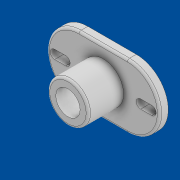
# Autodesk Inventor part: 부품1
Saved by Autodesk Inventor 2022 (Build 260153000, 153)
## iProperties
Created: 2022-09-19
Part Number: 부품1
Material: 일반
Document SubType Name: Modeling
Designer: USER
Density: 1 g/cm^3
Appearance: 기본값
Author: USER
Autodesk Inventor part; units mm, degrees
ref_plane "YZ Plane" through (0, 0, 0) normal (1, 0, 0) x (0, 1, 0)
ref_plane "XZ Plane" through (0, 0, 0) normal (0, 1, 0) x (-1, 0, 0)
sketch "스케치1" plane through (0, 0, 0) normal (0, 0, 1) x (1, 0, 0)
  line L0 (-22, 0) -> (22, 0) construction
  line L1 (-22, -29) -> (22, -29)
  line L2 (22, 29) -> (-22, 29)
  arc A0 (-22, 29) -> (-22, -29) centre (-22, 0) ccw
  arc A1 (22, -29) -> (22, 29) centre (22, 0) ccw
  line L3 (-44, 0) -> (-34, 0) construction
  line L4 (-44, -4) -> (-34, -4)
  line L5 (-34, 4) -> (-44, 4)
  arc A2 (-44, 4) -> (-44, -4) centre (-44, 0) ccw
  arc A3 (-34, -4) -> (-34, 4) centre (-34, 0) ccw
  line L6 (44, 0) -> (34, 0) construction
  line L7 (44, 4) -> (34, 4)
  line L8 (34, -4) -> (44, -4)
  arc A4 (44, -4) -> (44, 4) centre (44, 0) ccw
  arc A5 (34, 4) -> (34, -4) centre (34, 0) ccw
  circle A6 centre (0, 0) radius 18.5
  circle A7 centre (0, 0) radius 11
  point P0 (-39, 0)
  point P1 (39, 0)
  dimension "d0" = 29
  dimension "d1" = 102
  dimension "d2" = 10
  dimension "d3" = 8
  dimension "d4" = 10
  dimension "d5" = 8
  dimension "d6" = 68
  dimension "d7" = 34
  dimension "d8" = 37
  dimension "d9" = 22
  constraints: 24 end point, 12 point on circle, 12 tangent, 8 centre point, 3 coincident, 3 horizontal, 3 midpoint, 3 parallel
  measures "d0" radius of A1
  measures "d2" distance of L3.end L3.start
  measures "d3" distance between parallel lines of L5 L4
  measures "d4" distance of L6.start L6.end
  measures "d5" distance between parallel lines of L7 L8
  measures "d6" distance of L6.end L3.end
  measures "d7" distance of point (0, 0) L3.end
  measures "d8" diameter of A6
  measures "d9" diameter of A7
extrude "돌출1" add sketch "스케치1" along normal blind 8 contours A0 L2 A1 L1
extrude "돌출2" add sketch "스케치1" along normal blind 40 contours A6
ref_plane "작업 평면1" through (-22, 0, 0) normal (0, 1, 0) x (1, 0, 0)
sketch "스케치2" plane through (-22, 0, 0) normal (0, 1, 0) x (1, 0, 0)
  line L0 (36.5, 0) -> (34.1671, -19)
  line L1 (34.1671, -19) -> (9.8329, -19)
  line L2 (33, -40) -> (33, 0) projected
  line L3 (9.8329, -19) -> (7.5, 0)
  line L4 (85.0441, 0) -> (-77.2032, 0)
  line L5 (22, 10.7301) -> (22, -88.2666)
  point P0 (22, 0)
  point P1 (22, 0)
  point P2 (22, 0)
  point P3 (22, -19)
  dimension "d14" = 14
  dimension "d16" = 29
  dimension "d17" = 19
  dimension "d18" = 19
  dimension "d19" = 0
  dimension "d20" = 0
  dimension "d21" = 14.5
  constraints: 10 end point, 1 coincident, 1 horizontal, 1 perpendicular, 1 vertical
  measures "d14" angle of L3 L0
  measures "d16" distance of L3.end L0.start
  measures "d17" distance from line of L1 L0.start
  measures "d18" distance from line of L1 L3.end
  measures "d19" distance from line of L4 L3.end
  measures "d20" distance from line of point (22, 0) L4
  measures "d21" distance of L0.start point (22, 0)
revolve "회전1" cut sketch "스케치2" angle 360 about axis through (0, 0, -10.7301) along (0, 0, 1) contours L0 L1 L2 L4 | L2 L1 L5 L4
fillet "모깎기1" radius 2 1 edges at (-12.1671, 0, 19)
fillet "모깎기2" radius 2 5 edges at (-18.5, 0, 40) (0, -29, 8) (51, 0, 8) (0, 29, 8) (-51, 0, 8)
